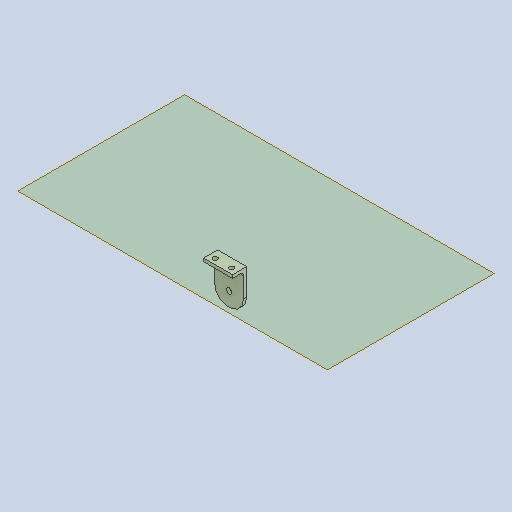
# Autodesk Inventor part: Soporte Motor
Saved by Autodesk Inventor 2023 (Build 270158000, 158)
## iProperties
Created: 2023-04-20
Part Number: Soporte Motor
Material: Genérico
Document SubType Name: Modeling
Designer: sergi
Density: 1 g/cm^3
Appearance: Valor por defecto
Author: sergi
Autodesk Inventor part; units mm, degrees
ref_plane "YZ Plane" through (0, 0, 0) normal (1, 0, 0) x (0, 1, 0)
ref_plane "XZ Plane" through (0, 0, 0) normal (0, 1, 0) x (-1, 0, 0)
ref_plane "XY Plane" through (0, 0, 0) normal (0, 0, 1) x (1, 0, 0)
sketch "Boceto1" plane through (0, 0, 0) normal (0, 0, 1) x (1, 0, 0)
  circle A0 centre (0, 0) radius 1.75
  circle A1 centre (0, 0) radius 9.25
  line L0 (43, 17) -> (-96.75, 17) projected
  line L1 (-9.25, 0) -> (-9.25, 17)
  line L2 (9.25, 0) -> (9.25, 17)
  dimension "d0" = 3.5
  dimension "d1" = 18.5
  constraints: 4 end point, 2 centre point, 2 coincident, 2 point on circle, 2 point on line, 1 perpendicular, 1 tangent, 1 vertical
  measures "d0" diameter of A0
  measures "d1" diameter of A1
extrude "Extrusión1" add sketch "Boceto1" along normal blind 2
ref_plane "Plano de trabajo1" through (83.25, 17, -70.5) normal (0, -1, 0) x (1, 0, 0)
sketch "Boceto3" plane through (83.25, 17, -70.5) normal (0, -1, 0) x (1, 0, 0)
  line L0 (-74, 72.5) -> (-92.5, 72.5) projected
  line L1 (-92.5, 72.5) -> (-74, 72.5)
  line L2 (-74, 72.5) -> (-74, 79.5)
  line L3 (-74, 79.5) -> (-92.5, 79.5)
  line L4 (-92.5, 79.5) -> (-92.5, 72.5)
  line L5 (-74, 76) -> (-78, 76)
  circle A0 centre (-78, 76) radius 1.5
  line L6 (-92.5, 76) -> (-88.5, 76)
  circle A1 centre (-88.5, 76) radius 1.5
  point P0 (-83.25, 70.5)
  dimension "d4" = 7
  dimension "d5" = 4
  dimension "d6" = 3
  dimension "d7" = 4
  dimension "d8" = 3
  constraints: 12 end point, 2 centre point, 2 coincident, 2 midpoint, 2 parallel, 1 horizontal, 1 perpendicular
  measures "d4" distance of L2.end L1.end
  measures "d5" distance of L5.start L5.end
  measures "d6" diameter of A0
  measures "d7" distance of L6.start L6.end
  measures "d8" diameter of A1
extrude "Extrusión2" add sketch "Boceto3" along normal blind 2
fillet "Empalme1" radius 2 1 edges at (0, 15, 2)
